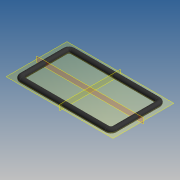
# Autodesk Inventor part: P020_Joint
Saved by Autodesk Inventor 2021.3 (Build 253353000, 353)
## iProperties
Created: 2021-11-12
Part Number: P020_Joint
Material: Rubber, Silicone
Document SubType Name: Modeling
Designer: gabri
Density: 1.25 g/cm^3
Appearance: Rubber - Black
Author: gabri
Autodesk Inventor part; units mm, degrees
sketch "Sketch2" plane through (0, 0, 0) normal (0, 0, 1) x (1, 0, 0)
  line L0 (29, -16.5) -> (-29, -16.5) construction
  line L1 (-29, -16.5) -> (-29, 16.5) construction
  line L2 (-29, 16.5) -> (29, 16.5) construction
  line L3 (29, 16.5) -> (29, -16.5) construction
  line L4 (29, -16.5) -> (-29, 16.5) construction
  line L5 (-29, -16.5) -> (29, 16.5) construction
  line L6 (25.5, -15) -> (-25.5, -15)
  line L7 (-27.5, -13) -> (-27.5, 13)
  line L8 (-25.5, 15) -> (25.5, 15)
  line L9 (27.5, 13) -> (27.5, -13)
  line L10 (27.5, -15) -> (-27.5, 15) construction
  line L11 (-27.5, -15) -> (27.5, 15) construction
  arc A0 (-25.5, 15) -> (-27.5, 13) centre (-25.5, 13) ccw
  arc A1 (-27.5, -13) -> (-25.5, -15) centre (-25.5, -13) ccw
  arc A2 (25.5, -15) -> (27.5, -13) centre (25.5, -13) ccw
  arc A3 (27.5, 13) -> (25.5, 15) centre (25.5, 13) ccw
  point P0 (0, 0)
  dimension "d0" = 58
  dimension "d1" = 33
  dimension "d9" = 1.5
  dimension "d10" = 1.5
  dimension "d14" = 2
  constraints: 24 end point, 8 point on circle, 8 point on line, 8 tangent, 4 centre point, 4 midpoint, 4 parallel, 3 equal radius, 2 horizontal, 2 perpendicular
  measures "d0" distance of L1.end L2.end
  measures "d1" distance of L0.end L1.end
  measures "d9" distance between parallel lines of L2 L8
  measures "d10" distance between parallel lines of L1 L7
  measures "d14" radius of A0
sketch "Sketch4" plane through (0, 0, 0) normal (1, 0, 0) x (0, 1, 0)
  line L0 (16.5, 0) -> (-16.5, 0) construction
  circle A0 centre (15, 0) radius 1.5
  point P0 (0, 0)
  dimension "d11" = 3
  constraints: 1 centre point, 1 coincident
  measures "d11" diameter of A0
sweep "Sweep1" add profiles "Sketch4" path "Sketch2" path curves L6 A2 L9 A3 L8 A0 L7 A1
body "Solid2"
